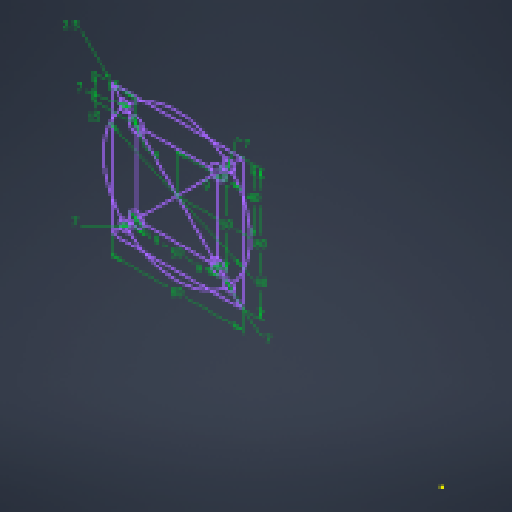
# Autodesk Inventor part: PL_TOP_1
Saved by Autodesk Inventor 2023 (Build 270158000, 158)
## iProperties
Created: 2025-09-04
Part Number: PL_TOP_1
Material: 일반
Document SubType Name: Modeling
Designer: k
Density: 1 g/cm^3
Appearance: 기본값
Author: k
Autodesk Inventor part; units mm, degrees
ref_plane "YZ Plane" through (0, 0, 0) normal (1, 0, 0) x (0, 1, 0)
ref_plane "XZ Plane" through (0, 0, 0) normal (0, 1, 0) x (-1, 0, 0)
ref_plane "XY Plane" through (0, 0, 0) normal (0, 0, 1) x (1, 0, 0)
sketch "스케치1" plane through (0, 0, 0) normal (0, 0, 1) x (1, 0, 0)
  line L0 (-199.6384, 113.7265) -> (-124.6384, 113.7265)
  line L1 (-122.1384, 111.2265) -> (-122.1384, 36.2265)
  line L2 (-124.6384, 33.7265) -> (-199.6384, 33.7265)
  line L3 (-202.1384, 36.2265) -> (-202.1384, 111.2265)
  circle A0 centre (-162.1384, 73.7265) radius 45
  line L4 (-122.1384, 113.7265) -> (-202.1384, 33.7265)
  line L5 (-202.1384, 113.7265) -> (-122.1384, 33.7265)
  circle A1 centre (-193.9582, 105.5463) radius 3.25
  circle A2 centre (-130.3186, 105.5463) radius 3.25
  circle A3 centre (-130.3186, 41.9067) radius 3.25
  circle A4 centre (-193.9582, 41.9067) radius 3.25
  line L6 (-187.1384, 98.7265) -> (-137.1384, 98.7265)
  line L7 (-137.1384, 98.7265) -> (-137.1384, 48.7265)
  line L8 (-137.1384, 48.7265) -> (-187.1384, 48.7265)
  line L9 (-187.1384, 48.7265) -> (-187.1384, 98.7265)
  circle A5 centre (-187.1384, 98.7265) radius 4.25
  circle A6 centre (-137.1384, 98.7265) radius 4.25
  circle A7 centre (-137.1384, 48.7265) radius 4.25
  circle A8 centre (-187.1384, 48.7265) radius 4.25
  arc A9 (-199.6384, 113.7265) -> (-202.1384, 111.2265) centre (-199.6384, 111.2265) ccw
  arc A10 (-202.1384, 36.2265) -> (-199.6384, 33.7265) centre (-199.6384, 36.2265) ccw
  arc A11 (-124.6384, 33.7265) -> (-122.1384, 36.2265) centre (-124.6384, 36.2265) ccw
  arc A12 (-122.1384, 111.2265) -> (-124.6384, 113.7265) centre (-124.6384, 111.2265) ccw
  circle A13 centre (-162.1384, 73.7265) radius 23.5
  point P0 (0, 0)
  dimension "d0" = 80
  dimension "d1" = 80
  dimension "d2" = 90
  dimension "d3" = 40
  dimension "d4" = 40
  dimension "d5" = 6.5
  dimension "d6" = 6.5
  dimension "d7" = 6.5
  dimension "d8" = 6.5
  dimension "d9" = 50
  dimension "d10" = 50
  dimension "d11" = 15
  dimension "d12" = 15
  dimension "d13" = 8.5
  dimension "d14" = 8.5
  dimension "d15" = 8.5
  dimension "d16" = 8.5
  dimension "d17" = 2.5
  dimension "d20" = 47
  constraints: 20 end point, 18 point on line, 14 centre point, 12 point on circle, 8 tangent, 4 parallel, 3 equal radius, 2 coincident, 2 horizontal, 2 perpendicular
  measures "d0" distance of L5.end L4.end
  measures "d1" distance of L4.start L5.end
  measures "d2" diameter of A0
  measures "d3" distance from line of L1 A0.centre
  measures "d4" distance from line of L0 A0.centre
  measures "d5" diameter of A1
  measures "d6" diameter of A2
  measures "d7" diameter of A3
  measures "d8" diameter of A4
  measures "d9" distance of L7.end L8.end
  measures "d10" distance of L6.end L7.end
  measures "d11" distance between parallel lines of L0 L6
  measures "d12" distance between parallel lines of L3 L9
  measures "d13" diameter of A5
  measures "d14" diameter of A6
  measures "d15" diameter of A7
  measures "d16" diameter of A8
  measures "d17" radius of A9
  measures "d20" diameter of A13
extrude "돌출1" add sketch "스케치1" along normal blind 6 contours L0 A0 A1 L5 A9 | L0 A0 A2 L4 A6 L6 A5 L5 A1 | L5 A1 A0 L3 A9 | L0 A12 L4 A2 A0 | A1 L5 A5 L9 A8 L4 A4 A0 L3 | A12 L1 A0 A2 L4 | A2 A0 L1 A3 L5 A7 L7 A6 L4 | A0 A4 L4 A10 L3 | A6 L4 A13 L5 A5 L6 | A5 L5 A13 L4 A8 L9 | L4 A4 A0 L2 A10 | L4 A8 L8 A7 L5 A3 A0 L2 A4 | L1 A11 L5 A3 A0 | A6 L7 A7 L5 A13 L4 | L4 A13 L5 A7 L8 A8 | A11 L2 A0 A3 L5
